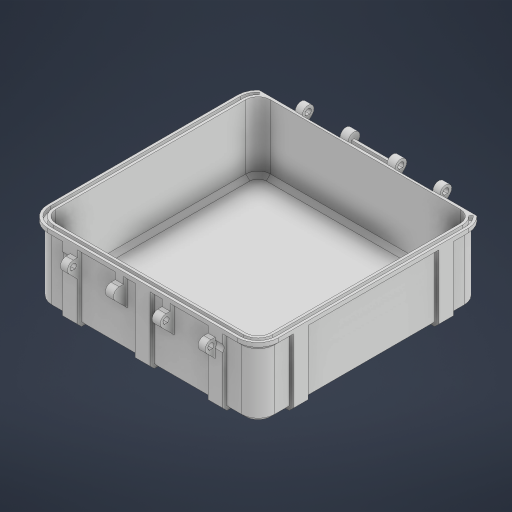
# Autodesk Inventor part: sumec_box_body
Saved by Autodesk Inventor 2024 (Build 280153000, 153)
## iProperties
Created: 2024-03-05
Part Number: sumec_box_body
Material: Všeobecné
Document SubType Name: Modeling
Designer: Simak
Density: 1 g/cm^3
Appearance: Výchozí
Author: Simak
Autodesk Inventor part; units mm, degrees
ref_plane "YZ Plane" through (0, 0, 0) normal (1, 0, 0) x (0, 1, 0)
ref_plane "XZ Plane" through (0, 0, 0) normal (0, 1, 0) x (-1, 0, 0)
ref_plane "XY Plane" through (0, 0, 0) normal (0, 0, 1) x (1, 0, 0)
sketch "velikost" plane through (0, 0, 0) normal (0, 1, 0) x (-1, 0, 0)
  line L0 (54.5, -54.5) -> (-54.5, -54.5)
  line L1 (-54.5, -54.5) -> (-54.5, 54.5)
  line L2 (-54.5, 54.5) -> (54.5, 54.5)
  line L3 (54.5, 54.5) -> (54.5, -54.5)
  line L4 (54.5, -54.5) -> (0, 0) construction
  line L5 (0, 0) -> (-54.5, -54.5) construction
  line L6 (0, 0) -> (-54.5, 54.5) construction
  dimension "d0" = 109
  dimension "d1" = 109
  constraints: 14 end point, 2 equal length, 2 parallel, 1 horizontal, 1 perpendicular
  measures "d0" distance of L0.start L0.end
  measures "d1" distance of L0.end L1.end
extrude "vyska" add sketch "velikost" along normal blind 35.5
fillet "Zaobleni_rohu" radius 8 4 edges at (-54.5, 17.75, 54.5) (54.5, 17.75, 54.5) (54.5, 17.75, -54.5) (-54.5, 17.75, -54.5)
shell "tloustka_sten" thickness 2 removed faces 1 at (15.5, 35.5, -12.8333)
sketch "vyztuhy-velikost" plane through (0, 35.5, 0) normal (0, 1, 0) x (1, 0, 0)
  arc A0 (-46.5, 52.5) -> (-52.5, 46.5) centre (-46.5, 46.5) ccw projected
  line L0 (-46.5, 52.5) -> (46.5, 52.5) projected
  arc A1 (52.5, 46.5) -> (46.5, 52.5) centre (46.5, 46.5) ccw projected
  line L1 (52.5, 46.5) -> (52.5, -46.5) projected
  arc A2 (46.5, -52.5) -> (52.5, -46.5) centre (46.5, -46.5) ccw projected
  line L2 (46.5, -52.5) -> (-46.5, -52.5) projected
  arc A3 (-52.5, -46.5) -> (-46.5, -52.5) centre (-46.5, -46.5) ccw projected
  line L3 (-52.5, -46.5) -> (-52.5, 46.5) projected
  arc A4 (-46.5, 54.5) -> (-54.5, 46.5) centre (-46.5, 46.5) ccw projected
  line L4 (-54.5, 46.5) -> (-54.5, -46.5) projected
  arc A5 (-54.5, -46.5) -> (-46.5, -54.5) centre (-46.5, -46.5) ccw projected
  line L5 (-46.5, -54.5) -> (46.5, -54.5) projected
  arc A6 (46.5, -54.5) -> (54.5, -46.5) centre (46.5, -46.5) ccw projected
  line L6 (54.5, -46.5) -> (54.5, 46.5) projected
  arc A7 (54.5, 46.5) -> (46.5, 54.5) centre (46.5, 46.5) ccw projected
  line L7 (46.5, 54.5) -> (-46.5, 54.5) projected
  line L8 (-39.2333, 54.5) -> (-39.2333, 56.5)
  line L9 (-39.2333, 56.5) -> (-31.9667, 56.5)
  line L10 (-31.9667, 56.5) -> (-31.9667, 54.5)
  line L11 (-3.6333, 54.5) -> (-3.6333, 56.5)
  line L12 (-3.6333, 56.5) -> (3.6333, 56.5)
  line L13 (3.6333, 56.5) -> (3.6333, 54.5)
  line L14 (31.9667, 54.5) -> (31.9667, 56.5)
  line L15 (31.9667, 56.5) -> (39.2333, 56.5)
  line L16 (39.2333, 56.5) -> (39.2333, 54.5)
  line L17 (46.5, 54.5) -> (-46.5, 54.5) projected
  line L18 (-3.6333, 56.5) -> (0, 54.5) construction
  line L19 (3.6333, 56.5) -> (0, 54.5) construction
  line L20 (-31.9667, 56.5) -> (-3.6333, 56.5) construction
  line L21 (3.6333, 56.5) -> (31.9667, 56.5) construction
  line L22 (-39.2333, 56.5) -> (-46.5, 56.5) construction
  line L23 (-46.5, 56.5) -> (-46.5, 54.5) construction
  line L24 (-52.5, 0) -> (52.5, 0)
  line L25 (0, 52.5) -> (0, -52.5)
  line L26 (46.5, -52.5) -> (-46.5, -52.5) projected
  line L27 (-54.5, -39.2333) -> (-56.5, -39.2333)
  line L28 (-56.5, -39.2333) -> (-56.5, -31.9667)
  line L29 (-56.5, -31.9667) -> (-54.5, -31.9667)
  line L30 (-54.5, 31.9667) -> (-56.5, 31.9667)
  line L31 (-56.5, 31.9667) -> (-56.5, 39.2333)
  line L32 (-56.5, 39.2333) -> (-54.5, 39.2333)
  line L33 (-56.5, -31.9667) -> (-56.5, 31.9667) construction
  line L34 (-56.5, -39.2333) -> (-56.5, -46.5) construction
  line L35 (-56.5, -46.5) -> (-54.5, -46.5) construction
  line L36 (-54.5, 46.5) -> (-54.5, -46.5) projected
  line L37 (-56.5, 39.2333) -> (-56.5, 46.5) construction
  line L38 (-56.5, 46.5) -> (-54.5, 46.5) construction
  line L39 (-54.5, 0) -> (-56.5, 31.9667) construction
  line L40 (-54.5, 0) -> (-56.5, -31.9667) construction
  line L41 (-39.2333, -54.5) -> (-39.2333, -56.5)
  line L42 (-39.2333, -56.5) -> (-31.9667, -56.5)
  line L43 (-31.9667, -56.5) -> (-31.9667, -54.5)
  line L44 (-3.6333, -54.5) -> (-3.6333, -56.5)
  line L45 (-3.6333, -56.5) -> (3.6333, -56.5)
  line L46 (3.6333, -56.5) -> (3.6333, -54.5)
  line L47 (31.9667, -54.5) -> (31.9667, -56.5)
  line L48 (31.9667, -56.5) -> (39.2333, -56.5)
  line L49 (39.2333, -56.5) -> (39.2333, -54.5)
  line L50 (46.5, -54.5) -> (-46.5, -54.5)
  line L51 (-3.6333, -56.5) -> (0, -54.5) construction
  line L52 (3.6333, -56.5) -> (0, -54.5) construction
  line L53 (-31.9667, -56.5) -> (-3.6333, -56.5) construction
  line L54 (3.6333, -56.5) -> (31.9667, -56.5) construction
  line L55 (-39.2333, -56.5) -> (-46.5, -56.5) construction
  line L56 (-46.5, -56.5) -> (-46.5, -54.5) construction
  line L57 (54.5, 46.5) -> (54.5, -46.5)
  line L58 (56.5, -31.9667) -> (56.5, 31.9667) construction
  line L59 (54.5, -39.2333) -> (56.5, -39.2333)
  line L60 (56.5, -39.2333) -> (56.5, -46.5) construction
  line L61 (56.5, -31.9667) -> (54.5, -31.9667)
  line L62 (56.5, -46.5) -> (54.5, -46.5) construction
  line L63 (56.5, -39.2333) -> (56.5, -31.9667)
  line L64 (56.5, 31.9667) -> (56.5, 39.2333)
  line L65 (56.5, 39.2333) -> (54.5, 39.2333)
  line L66 (54.5, 31.9667) -> (56.5, 31.9667)
  line L67 (54.5, 46.5) -> (54.5, -46.5)
  line L68 (56.5, 39.2333) -> (56.5, 46.5) construction
  line L69 (56.5, 46.5) -> (54.5, 46.5) construction
  line L70 (54.5, 0) -> (56.5, 31.9667) construction
  line L71 (54.5, 0) -> (56.5, -31.9667) construction
  point P0 (0, 0)
  point P1 (54.5, 39.2333)
  point P2 (54.5, 31.9667)
  point P3 (54.5, -31.9667)
  point P4 (54.5, -39.2333)
  point P5 (39.2333, -54.5)
  point P6 (31.9667, -54.5)
  point P7 (3.6333, -54.5)
  point P8 (-3.6333, -54.5)
  point P9 (-31.9667, -54.5)
  point P10 (-39.2333, -54.5)
  point P11 (-54.5, -39.2333)
  point P12 (-54.5, -31.9667)
  point P13 (-54.5, 31.9667)
  point P14 (-54.5, 39.2333)
  dimension "d5" = 2
  dimension "d6" = 2
  dimension "d7" = 7.2667
  dimension "d8" = 2
  constraints: 120 end point, 25 symmetric about line, 20 point on line, 14 equal length, 11 perpendicular, 5 midpoint, 5 vertical, 2 horizontal, 5 other
  measures "d6" distance of L9.end L10.end
  measures "d7" distance of L11.end L12.end
  measures "d8" distance of L33.start L29.end
extrude "vyztuhy" add sketch "vyztuhy-velikost" against normal up to surface (35.5 mm away) contours L8 L9 L10 L7 | L4 L30 L31 L32 | L11 L12 L13 L7 | L4 L27 L28 L29 | L14 L15 L16 L7 | L5 L43 L42 L41 | L65 L64 L66 L6 | L5 L46 L45 L44 | L61 L63 L59 L6 | L5 L49 L48 L47
chamfer "Zkoseni_spodku" distance 2 angle 45 36 edges at (-17.8, 0, 54.5) (17.8, 0, 54.5) (0, 0, 56.5) (35.6, 0, 56.5) (42.8667, 0, 54.5) (52.1569, 0, 52.1569) (54.5, 0, 42.8667) (56.5, 0, 35.6) (54.5, 0, 0) (56.5, 0, -35.6) (52.1569, 0, -52.1569) (42.8667, 0, -54.5) (54.5, 0, -42.8667) (35.6, 0, -56.5) (17.8, 0, -54.5) (0, 0, -56.5) (-17.8, 0, -54.5) (-35.6, 0, -56.5) (-42.8667, 0, -54.5) (-52.1569, 0, -52.1569) (-54.5, 0, -42.8667) (-56.5, 0, -35.6) (-54.5, 0, 0) (-56.5, 0, 35.6) (-54.5, 0, 42.8667) (-52.1569, 0, 52.1569) (-42.8667, 0, 54.5) (-35.6, 0, 56.5) (-52.5, 2, 0) (-50.7426, 2, 50.7426) (0, 2, 52.5) (50.7426, 2, 50.7426) (52.5, 2, 0) (50.7426, 2, -50.7426) (0, 2, -52.5) (-50.7426, 2, -50.7426)
sketch "Náčrt4" plane through (39.2333, 35.5, -54.5) normal (1, 0, 0) x (0, 0, -1)
  line L0 (-2, 0) -> (-2, -31.5) projected
  line L1 (2, 0) -> (2, -33.5) projected
  line L2 (-8, 0) -> (0, 0) projected
  line L3 (-0.75, 0) -> (-0.75, -2)
  line L4 (-0.75, -2) -> (0.75, -2)
  line L5 (0.75, -2) -> (0.75, 0)
  line L6 (-0.75, -2) -> (-2, -2) construction
  line L7 (0.75, -2) -> (2, -2) construction
  line L8 (2, 0) -> (0, 0) projected
  line L9 (2, -4) -> (-2, -4)
  point P0 (-54.5, -35.5)
  dimension "d16" = 1.5
  dimension "d17" = 2
  dimension "d18" = 2
  constraints: 12 end point, 7 point on line, 5 perpendicular, 1 collinear
  measures "d16" distance of L3.end L4.end
  measures "d17" distance between parallel lines of L8 L4
  measures "d18" distance between parallel lines of L9 L4
sketch "Náčrt3" plane through (0, 35.5, 0) normal (0, 1, 0) x (1, 0, 0)
  arc A0 (-46.5, 52.5) -> (-52.5, 46.5) centre (-46.5, 46.5) ccw projected
  line L0 (-46.5, 52.5) -> (46.5, 52.5) projected
  arc A1 (52.5, 46.5) -> (46.5, 52.5) centre (46.5, 46.5) ccw projected
  line L1 (52.5, 46.5) -> (52.5, -46.5) projected
  arc A2 (46.5, -52.5) -> (52.5, -46.5) centre (46.5, -46.5) ccw projected
  line L2 (46.5, -52.5) -> (-46.5, -52.5) projected
  arc A3 (-52.5, -46.5) -> (-46.5, -52.5) centre (-46.5, -46.5) ccw projected
  line L3 (-52.5, -46.5) -> (-52.5, 46.5) projected
  arc A4 (-46.5, 54.5) -> (-54.5, 46.5) centre (-46.5, 46.5) ccw projected
  line L4 (-54.5, 46.5) -> (-54.5, 39.2333) projected
  line L5 (-56.5, 31.9667) -> (-54.5, 31.9667) projected
  line L6 (-54.5, 31.9667) -> (-54.5, -31.9667) projected
  arc A5 (-54.5, -46.5) -> (-46.5, -54.5) centre (-46.5, -46.5) ccw projected
  line L7 (-46.5, -54.5) -> (-39.2333, -54.5) projected
  line L8 (-39.2333, -54.5) -> (-39.2333, -56.5) projected
  line L9 (-39.2333, -56.5) -> (-31.9667, -56.5) projected
  line L10 (-31.9667, -56.5) -> (-31.9667, -54.5) projected
  line L11 (-31.9667, -54.5) -> (-3.6333, -54.5) projected
  line L12 (-3.6333, -54.5) -> (-3.6333, -56.5) projected
  line L13 (-3.6333, -56.5) -> (3.6333, -56.5) projected
  line L14 (3.6333, -56.5) -> (3.6333, -54.5) projected
  line L15 (3.6333, -54.5) -> (31.9667, -54.5) projected
  line L16 (31.9667, -54.5) -> (31.9667, -56.5) projected
  line L17 (31.9667, -56.5) -> (39.2333, -56.5) projected
  line L18 (39.2333, -56.5) -> (39.2333, -54.5) projected
  line L19 (39.2333, -54.5) -> (46.5, -54.5) projected
  arc A6 (46.5, -54.5) -> (54.5, -46.5) centre (46.5, -46.5) ccw projected
  line L20 (54.5, -46.5) -> (54.5, -39.2333) projected
  line L21 (56.5, -31.9667) -> (54.5, -31.9667) projected
  line L22 (54.5, -31.9667) -> (54.5, 31.9667) projected
  arc A7 (54.5, 46.5) -> (46.5, 54.5) centre (46.5, 46.5) ccw projected
  line L23 (46.5, 54.5) -> (39.2333, 54.5) projected
  line L24 (39.2333, 54.5) -> (39.2333, 56.5) projected
  line L25 (39.2333, 56.5) -> (31.9667, 56.5) projected
  line L26 (31.9667, 56.5) -> (31.9667, 54.5) projected
  line L27 (31.9667, 54.5) -> (3.6333, 54.5) projected
  line L28 (3.6333, 54.5) -> (3.6333, 56.5) projected
  line L29 (3.6333, 56.5) -> (-3.6333, 56.5) projected
  line L30 (-3.6333, 56.5) -> (-3.6333, 54.5) projected
  line L31 (-3.6333, 54.5) -> (-31.9667, 54.5) projected
  line L32 (-31.9667, 54.5) -> (-31.9667, 56.5) projected
  line L33 (-31.9667, 56.5) -> (-39.2333, 56.5) projected
  line L34 (-39.2333, 56.5) -> (-39.2333, 54.5) projected
  line L35 (-39.2333, 54.5) -> (-46.5, 54.5) projected
  line L36 (-54.5, -31.9667) -> (-56.5, -31.9667) projected
  line L37 (-56.5, -31.9667) -> (-56.5, -39.2333) projected
  line L38 (54.5, 31.9667) -> (56.5, 31.9667) projected
  line L39 (56.5, 31.9667) -> (56.5, 39.2333) projected
  line L40 (-54.5, 39.2333) -> (-56.5, 39.2333) projected
  line L41 (-56.5, 39.2333) -> (-56.5, 31.9667) projected
  line L42 (-56.5, -39.2333) -> (-54.5, -39.2333) projected
  line L43 (-54.5, -39.2333) -> (-54.5, -46.5) projected
  line L44 (54.5, -39.2333) -> (56.5, -39.2333) projected
  line L45 (56.5, -39.2333) -> (56.5, -31.9667) projected
  line L46 (56.5, 39.2333) -> (54.5, 39.2333) projected
  line L47 (54.5, 39.2333) -> (54.5, 46.5) projected
  point P0 (0, 0)
sweep "tesnici_drazka" add profiles "Náčrt4" path "Náčrt3" path curves L0 A0 L3 A3 L2 A2 L1 A1 contours L2 L3 L4 L5 L8 L1 L9 L0
sweep "tesnici_drazka-zahloubeni" cut profiles "Náčrt4" path "Náčrt3" path curves L0 A0 L3 A3 L2 A2 L1 A1 contours L2 L8 L5 L4 L3
chamfer "tesnici_drazka-zkoseni" distance 2 angle 45 18 edges at (53.5711, 31.5, -53.5711) (42.8667, 31.5, -56.5) (56.5, 31.5, -42.8667) (17.8, 31.5, -56.5) (-17.8, 31.5, -56.5) (56.5, 31.5, 0) (56.5, 31.5, 42.8667) (53.5711, 31.5, 53.5711) (42.8667, 31.5, 56.5) (-53.5711, 31.5, -53.5711) (-56.5, 31.5, -42.8667) (-42.8667, 31.5, -56.5) (-56.5, 31.5, 0) (-53.5711, 31.5, 53.5711) (-42.8667, 31.5, 56.5) (-56.5, 31.5, 42.8667) (17.8, 31.5, 56.5) (-17.8, 31.5, 56.5)
sketch "pant-main_nacrt" plane through (31.9667, 0, -54.5) normal (-1, 0, 0) x (0, 0, 1)
  line L0 (0, 2) -> (0, 31.5) projected
  line L1 (2, 0) -> (0, 2) projected
  line L2 (0, 0) -> (2, 0) projected
  line L3 (-2, 2) -> (0, 0) projected
  line L4 (-2, 33.5) -> (-2, 2) projected
  line L5 (0, 31.5) -> (-2, 33.5) projected
  circle A0 centre (-2, 35.5) radius 1.55
  circle A1 centre (-2, 35.5) radius 2.875
  line L6 (-4.0329, 33.4671) -> (-2, 31.4341)
  line L7 (-2, 31.4341) -> (0, 29.4341)
  line L8 (8, 33.5) -> (-2, 33.5) projected
  line L9 (8, 35.5) -> (8, 33.5) projected
  line L10 (-2, 35.5) -> (8, 35.5) projected
  line L11 (-2, 35.5) -> (-2, 33.5) projected
  line L12 (8, 31.5) -> (8, 33.5) projected
  line L13 (8, 33.5) -> (-2, 33.5) projected
  line L14 (0, 31.5) -> (-2, 33.5) projected
  line L15 (8, 31.5) -> (0, 31.5) projected
  line L16 (0.75, 33.5) -> (0.75, 35.5) projected
  line L17 (0.75, 33.5) -> (8, 33.5) projected
  line L18 (8, 33.5) -> (8, 35.5) projected
  line L19 (0.75, 35.5) -> (8, 35.5) projected
  line L20 (2, 35.5) -> (2, 4) projected
  circle A2 centre (-2, 35.5) radius 3.025
  circle A3 centre (-2, 35.5) radius 2.7
  point P0 (54.5, 0)
  point P1 (-2, 30)
  point P2 (0.875, 35.5)
  point P3 (-2, 32.625)
  point P4 (-1.23, 32.73)
  point P5 (0.0653, 33.5)
  point P6 (-2, 33.5)
  point P7 (-0.45, 35.5)
  point P8 (-2, 33.95)
  point P9 (0.75, 33.5)
  point P10 (0.75, 34.2398)
  point P11 (1.025, 35.5)
  point P12 (-1.1092, 32.6092)
  point P13 (-2, 32.475)
  point P14 (0.2695, 33.5)
  dimension "d28" = 5.75
  dimension "d27" = 3.1
  dimension "d71" = 0.15
  dimension "d78" = 5.4
  constraints: 4 end point, 3 centre point, 3 coincident, 2 point on line, 1 collinear, 1 parallel, 4 other
  measures "d27" diameter of A0
  measures "d78" diameter of A3
extrude "Vysunutí3" cut sketch "pant-main_nacrt" along normal blind 22 and the other way blind 3.5 contours A2 L4 A1 L5 | L5 A1 L8 A2 | A2 L6 A1 L4 | A2 L10 A1 L6 | A1 L4 A3 L5 | L5 A3 L8 A1 | L8 A1 L16 A2 | A1 L10 A3 L4 | A2 L16 A1 L10 | A3 L4 L5 | L5 L8 A3 | L8 A3 L10 L16 A1 | A3 L10 A0 L11 L4 | A1 L16 L10 | L11 A0 L10 A3 L8 | L11 L10 A0 | A0 L10 L11
extrude "Vysunutí18" cut sketch "pant-main_nacrt" against normal through all contours A3 L4 L5 | L5 L8 A3 | A3 L10 A0 L11 L4 | L11 A0 L10 A3 L8 | L11 L10 A0 | A0 L10 L11
extrude "Vysunutí4" add sketch "pant-main_nacrt" against normal blind 3.5 contours L6 A2 L4 | A2 L4 A1 L5 | L5 A1 L8 A2 | A2 L6 A1 L4 | A1 L4 A3 L5 | L5 A3 L8 A1 | A2 L16 L8 | L8 A1 L16 A2 | A1 L10 A3 L4 | A2 L16 A1 L10 | A3 L4 L5 | L5 L8 A3 | L8 A3 L10 L16 A1 | A3 L10 A0 L11 L4 | A1 L16 L10 | L11 A0 L10 A3 L8
extrude "Vysunutí19" add sketch "pant-main_nacrt" along normal up to surface (31.9667 mm away) contours A2 L16 L8
sketch "Náčrt13" plane through (31.9667, 0, -54.5) normal (-1, 0, 0) x (0, 0, 1)
  circle A0 centre (-2, 35.5) radius 1.55 projected
  line L0 (0.75, 35.5) -> (0.875, 35.5) projected
  line L1 (0.75, 33.5) -> (0.75, 35.5) projected
  line L2 (-0.1862, 33.5) -> (0.75, 33.5) projected
  arc A1 (-2, 32.8) -> (-0.1862, 33.5) centre (-2, 35.5) ccw projected
  line L3 (-2, 31.4341) -> (-2, 32.8) projected
  line L4 (-2, 31.4341) -> (-4.0329, 33.4671) projected
  arc A2 (0.875, 35.5) -> (-4.0329, 33.4671) centre (-2, 35.5) ccw projected
  line L5 (-2.75, 34.1435) -> (-2.75, 34.3)
  line L6 (-2.75, 34.3) -> (-1.25, 34.3)
  line L7 (-1.25, 34.3) -> (-1.25, 34.1435)
  point P0 (54.5, 0)
  dimension "d83" = 2.75
  dimension "d84" = 1.5
  constraints: 6 end point, 2 perpendicular, 2 point on circle, 1 parallel, 1 vertical
  measures "d84" distance of L5.end L6.end
extrude "Vysunutí20" add sketch "Náčrt13" against normal up to surface (3.5 mm away) contours L5 L6 L7 A0 picked at (-2.0521, 34.186)
ref_plane "Pracovní rovina1" through (13.4667, 0, -54.5) normal (-1, 0, 0) x (0, 0, 1)
sketch "Náčrt14" plane through (13.4667, 0, -54.5) normal (-1, 0, 0) x (0, 0, 1)
  arc A0 (-1.1092, 32.6092) -> (1.025, 35.5) centre (-2, 35.5) ccw projected
  line L0 (1.025, 35.5) -> (0.875, 35.5) projected
  arc A1 (0.875, 35.5) -> (-4.0329, 33.4671) centre (-2, 35.5) ccw projected
  line L1 (-4.0329, 33.4671) -> (-2, 31.4341) projected
  line L2 (-2, 31.4341) -> (-2, 2) projected
  line L3 (0, 0) -> (-2, 2) projected
  line L4 (2, 0) -> (0, 0) projected
  line L5 (0, 2) -> (2, 0) projected
  line L6 (0, 31.5) -> (0, 2) projected
  line L7 (-1.1092, 32.6092) -> (0, 31.5) projected
  arc A2 (-1.25, 34.1435) -> (-2.75, 34.1435) centre (-2, 35.5) ccw projected
  line L8 (-1.25, 34.1435) -> (-1.25, 34.3) projected
  line L9 (-1.25, 34.3) -> (-2.75, 34.3) projected
  line L10 (-2.75, 34.3) -> (-2.75, 34.1435) projected
  line L11 (-2, 31.4341) -> (0, 29.4341)
  point P0 (54.5, 0)
  constraints: 2 end point, 1 collinear, 1 point on line
extrude "Vysunutí21" add sketch "Náčrt14" along normal up to surface (3.5 mm away) contours L7 L6 L11 L1 A1 L0 A0
sketch "Náčrt15" plane through (9.9667, 29.4341, -54.5) normal (-1, 0, 0) x (0, 0, 1)
  line L0 (0.875, 6.0659) -> (0.75, 6.0659) projected
  arc A0 (0.875, 6.0659) -> (-4.0329, 4.0329) centre (-2, 6.0659) ccw projected
  line L1 (0, 0) -> (-4.0329, 4.0329) projected
  line L2 (-2, 4.8659) -> (-2, 4.0659) projected
  line L3 (-2.75, 4.8659) -> (-2, 4.8659) projected
  line L4 (-2.75, 4.7094) -> (-2.75, 4.8659) projected
  arc A1 (-0.75, 5.1493) -> (-2.75, 4.7094) centre (-2, 6.0659) ccw projected
  line L5 (-0.75, 4.0659) -> (-0.75, 5.1493) projected
  line L6 (0.2695, 4.0659) -> (-0.75, 4.0659) projected
  line L7 (0.75, 6.0659) -> (0.75, 4.8057) projected
  arc A2 (-1.1092, 3.175) -> (1.025, 6.0659) centre (-2, 6.0659) ccw projected
  line L8 (-1.1092, 3.175) -> (0, 2.0659) projected
  arc A3 (0.2695, 4.0659) -> (0.75, 4.8057) centre (-2, 6.0659) ccw projected
  line L9 (0, 2.0659) -> (0, 0) projected
  line L10 (-2, 4.0659) -> (0, 2.0659) projected
  point P0 (54.5, -29.4341)
  point P1 (0.2695, 4.0659)
  point P2 (0.75, 4.8057)
extrude "Vysunutí22" add sketch "Náčrt15" along normal blind 0.5 contours L0 L7 A2 L6 L5 A1 L4 L3 L2 L10 L8 L9 L1 A0
sketch "Náčrt16" plane through (31.9667, 2, -54.5) normal (0, 0, -1) x (-1, 0, 0)
  line L0 (18.5, 30.6092) -> (18.5, 33.5) projected
  line L1 (0, 33.5) -> (18.5, 33.5) projected
  line L2 (0, 33.5) -> (0, 30.6092) projected
  line L3 (18.5, 30.6092) -> (0, 30.6092) projected
  line L4 (18.5, 30.6092) -> (0, 30.6092) projected
  line L5 (0, 30.6092) -> (0, 29.5) projected
  line L6 (18.5, 29.5) -> (0, 29.5) projected
  line L7 (22.5, 27.4341) -> (18.5, 27.4341) projected
  line L8 (18.5, 29.5) -> (0, 29.5) projected
  line L9 (0, 29.5) -> (0, 0) projected
  line L10 (28.3333, 0) -> (0, 0) projected
  line L11 (28.3333, 0) -> (28.3333, 29.5) projected
  line L12 (63.9333, 29.5) -> (35.6, 29.5) projected
  line L13 (35.6, 29.5) -> (35.6, 0) projected
  line L14 (63.9333, 0) -> (35.6, 0) projected
  line L15 (63.9333, 0) -> (63.9333, 29.5) projected
  line L16 (18.5, 29.5) -> (18.5, 30.6092) projected
  line L17 (18.5, 27.4341) -> (18.5, 29.5) projected
  line L18 (22.5, 29.5) -> (22.5, 27.4341) projected
  line L19 (28.3333, 29.5) -> (22.5, 29.5) projected
  point P0 (31.9667, -2)
extrude "Vysunutí23" cut sketch "Náčrt16" along normal through all contours L3 L2 L1 L0 | L16 L6 L5 L3
sketch "Náčrt17" plane through (35.4667, 0, -54.5) normal (1, 0, 0) x (0, 0, -1)
  arc A0 (2.75, 34.1435) -> (1.25, 34.1435) centre (2, 35.5) ccw projected
  line L0 (2.75, 34.1435) -> (2.75, 34.3) projected
  line L1 (2.75, 34.3) -> (1.25, 34.3) projected
  line L2 (1.25, 34.3) -> (1.25, 34.1435) projected
  line L3 (-0.75, 35.5) -> (-0.875, 35.5) projected
  line L4 (-0.75, 33.5) -> (-0.75, 35.5) projected
  line L5 (0.1862, 33.5) -> (-0.75, 33.5) projected
  arc A1 (0.1862, 33.5) -> (2, 32.8) centre (2, 35.5) ccw projected
  line L6 (2, 31.4341) -> (2, 32.8) projected
  line L7 (2, 31.4341) -> (4.0329, 33.4671) projected
  arc A2 (4.0329, 33.4671) -> (-0.875, 35.5) centre (2, 35.5) ccw projected
  spline S0 degree 6 poles (0.1863, 33.4999) (0.1273, 33.5533) (0.0685, 33.6105) (0.0102, 33.6714) (-0.0473, 33.7362) (-0.1036, 33.805) (-0.193, 33.9239) (-0.227, 33.9717) (-0.2603, 34.021) (-0.2927, 34.0719) (-0.3241, 34.1243) (-0.3771, 34.2188) (-0.3992, 34.2602) (-0.4207, 34.3024) (-0.4414, 34.3454) (-0.4613, 34.3891) (-0.5499, 34.5952) (-0.6084, 34.766) (-0.6538, 34.9443) (-0.6846, 35.1278) (-0.7, 35.314) (-0.7, 35.5) knots 0 0 0 0 0 0 0 0.258993 0.258993 0.258993 0.258993 0.258993 0.423699 0.423699 0.423699 0.423699 0.423699 0.547895 0.547895 0.547895 0.547895 0.547895 1 1 1 1 1 1 1 projected
  line L8 (-0.7, 35.5) -> (-8, 35.5) projected
  point P0 (-54.5, 0)
  constraints: 1 other
extrude "Vysunutí24" add sketch "Náčrt17" along normal up to next contours L8 S0 L5 L4
sketch "Náčrt18" plane through (0, 35.5, 0) normal (0, 1, 0) x (1, 0, 0)
  arc A0 (55.25, 46.5) -> (51.399, 53.75) centre (46.5, 46.5) ccw projected
  arc A1 (53.75, 46.5) -> (46.5, 53.75) centre (46.5, 46.5) ccw projected
  line L0 (46.5, 46.5) -> (52.3577, 53)
  line L1 (46.5, 53.75) -> (51.399, 53.75) projected
  line L2 (53.3345, 53.8) -> (35.4667, 53.8) projected
  point P0 (0, 0)
  point P1 (51.3535, 51.8857)
  dimension "d99" = 0.8
  constraints: 2 end point, 1 point on circle
  measures "d99" distance from line of L2 L0.end
extrude "Vysunutí25" add sketch "Náčrt18" against normal up to next
sketch "Náčrt19" plane through (9.9667, 0, -54.5) normal (1, 0, 0) x (0, 0, -1)
  arc A0 (4.0329, 33.4671) -> (-0.875, 35.5) centre (2, 35.5) ccw projected
  line L0 (-1.025, 35.5) -> (-0.875, 35.5) projected
  arc A1 (-1.025, 35.5) -> (0, 33.2305) centre (2, 35.5) ccw projected
  line L1 (4.0329, 33.4671) -> (0, 29.4341) projected
  arc A2 (2.75, 34.1435) -> (1.25, 34.1435) centre (2, 35.5) ccw projected
  line L2 (2.75, 34.3) -> (2.75, 34.1435) projected
  line L3 (1.25, 34.3) -> (2.75, 34.3) projected
  line L4 (1.25, 34.1435) -> (1.25, 34.3) projected
  line L5 (0, 29.4341) -> (0, 33.2305) projected
  point P0 (-54.5, 0)
extrude "Vysunutí26" add sketch "Náčrt19" against normal up to surface (0.5 mm away) contours L2 L3 L4 A2
mirror "pant-zrcadleni" about plane through (0, 0, 0) normal (1, 0, 0) of "Vysunutí3", "Vysunutí4", "Vysunutí24", "Vysunutí25", "Vysunutí23", "Vysunutí22", "Vysunutí21", "Vysunutí19", "Vysunutí20", "Vysunutí18", "Vysunutí26"
sketch "latch-main_nacrt" plane through (31.9667, 0, 52.5) normal (-1, 0, 0) x (0, 0, 1)
  line L0 (4, 33.5) -> (4, 2) projected
  line L1 (2, 0) -> (4, 2) projected
  line L2 (0, 0) -> (2, 0) projected
  line L3 (2, 2) -> (0, 0) projected
  line L4 (2, 31.5) -> (2, 2) projected
  line L5 (4, 33.5) -> (2, 31.5) projected
  line L6 (4, 35.5) -> (-6, 35.5) projected
  line L7 (2.75, 33.5) -> (-6, 33.5) projected
  line L8 (1.25, 33.5) -> (1.25, 35.5) projected
  line L9 (2.75, 33.5) -> (2.75, 35.5) projected
  line L10 (4, 35.5) -> (4, 33.5) projected
  circle A0 centre (6.05, 27.3) radius 1.55
  line L11 (5.3, 25.9435) -> (5.3, 26.1)
  line L12 (5.3, 26.1) -> (6.8, 26.1)
  line L13 (6.8, 26.1) -> (6.8, 25.9435)
  circle A1 centre (6.05, 27.3) radius 2.875
  line L14 (6.05, 30.175) -> (2, 30.175)
  line L15 (2, 19.1841) -> (8.0829, 25.2671)
  circle A2 centre (6.05, 27.3) radius 2.7
  point P0 (-52.5, 0)
  point P1 (4, 29.3157)
  point P2 (4, 25.2843)
  dimension "d52" = 3.1
  dimension "d53" = 8.2
  dimension "d54" = 4.05
  dimension "d55" = 2.75
  dimension "d56" = 1.5
  dimension "d57" = 5.75
  dimension "d58" = 45
  dimension "d63" = 5.4
  constraints: 10 end point, 4 point on circle, 3 centre point, 3 perpendicular, 2 coincident, 2 point on line, 2 tangent, 1 parallel, 1 vertical
  measures "d52" diameter of A0
  measures "d53" distance from line of L6 A0.centre
  measures "d54" distance from line of L4 A0.centre
  measures "d56" distance of L11.end L12.end
  measures "d57" diameter of A1
  measures "d58" angle of L4 L15
  measures "d63" diameter of A2
extrude "Vysunutí14" cut sketch "latch-main_nacrt" against normal up to next contours A2 L0 | L0 A2
extrude "Vysunutí12" add sketch "latch-main_nacrt" against normal blind 3.5 contours L14 A1 L0 | L0 A1 L15 L4 L14 | A1 L0 A2 | L0 A2 A1 | A2 L0 | L0 A2 | A1 L15 L0 | L11 L12 L13 A0 picked at (5.9979, 25.986)
ref_plane "Pracovní rovina3" through (13.4667, 0, 52.5) normal (-1, 0, 0) x (0, 0, 1)
sketch "Náčrt10" plane through (13.4667, 0, 52.5) normal (-1, 0, 0) x (0, 0, 1)
  arc A0 (6.8, 25.9435) -> (5.3, 25.9435) centre (6.05, 27.3) ccw projected
  line L0 (6.8, 25.9435) -> (6.8, 26.1) projected
  line L1 (6.8, 26.1) -> (5.3, 26.1) projected
  line L2 (5.3, 26.1) -> (5.3, 25.9435) projected
  line L3 (4, 21.1841) -> (8.0829, 25.2671) projected
  arc A1 (8.0829, 25.2671) -> (6.05, 30.175) centre (6.05, 27.3) ccw projected
  line L4 (6.05, 30.175) -> (4, 30.175) projected
  line L5 (4, 33.5) -> (4, 30.175) projected
  line L6 (2, 31.5) -> (4, 33.5) projected
  line L7 (2, 2) -> (2, 31.5) projected
  line L8 (0, 0) -> (2, 2) projected
  line L9 (2, 0) -> (0, 0) projected
  line L10 (4, 2) -> (2, 0) projected
  line L11 (4, 21.1841) -> (4, 2) projected
  line L12 (4, 30.175) -> (2, 30.175)
  line L13 (4, 21.1841) -> (2, 19.1841)
  line L14 (4, 30.175) -> (2, 31.5)
  point P0 (-52.5, 0)
  constraints: 6 end point, 2 collinear, 2 point on line
extrude "Vysunutí15" add sketch "Náčrt10" along normal blind 4 contours L13 L7 L12 L4 A1 L3 | L7 L14 L12 | L14 L6 L5
sketch "Náčrt12" plane through (9.4667, 0, 52.5) normal (-1, 0, 0) x (0, 0, 1)
  line L0 (2, 19.1841) -> (8.0829, 25.2671) projected
  arc A0 (8.0829, 25.2671) -> (6.05, 30.175) centre (6.05, 27.3) ccw projected
  line L1 (6.05, 30.175) -> (4, 30.175) projected
  line L2 (6.8, 26.1) -> (5.3, 26.1) projected
  line L3 (5.3, 26.1) -> (5.3, 25.9435) projected
  arc A1 (6.8, 25.9435) -> (5.3, 25.9435) centre (6.05, 27.3) ccw projected
  line L4 (6.8, 25.9435) -> (6.8, 26.1) projected
  line L5 (4, 30.175) -> (4, 33.5) projected
  line L6 (2, 31.5) -> (4, 33.5) projected
  line L7 (2, 19.1841) -> (2, 31.5) projected
  point P0 (-52.5, 0)
extrude "Vysunutí16" add sketch "Náčrt12" against normal blind 0.5 contours L2 L3 A1 L4
mirror "latch-zrcadleni" about plane through (0, 0, 0) normal (1, 0, 0) of "Vysunutí16", "Vysunutí14", "Vysunutí12", "Vysunutí15"
fillet "Zaoblení2" radius 1 8 edges at (42.8667, 32.8736, -55.8737) (49.4352, 32.9845, -55.519) (53.0393, 34.3323, -54.0656) (37.35, 32.8, -56.5) (-37.35, 32.8, -56.5) (-49.4352, 32.9845, -55.519) (-42.8667, 32.8736, -55.8737) (-53.0393, 34.3323, -54.0656)
ref_plane "Pracovní rovina2" through (-13.4667, 0, -54.5) normal (-1, 0, 0) x (0, 0, 1)
ref_plane "Pracovní rovina4" through (-13.4667, 0, 52.5) normal (-1, 0, 0) x (0, 0, 1)
